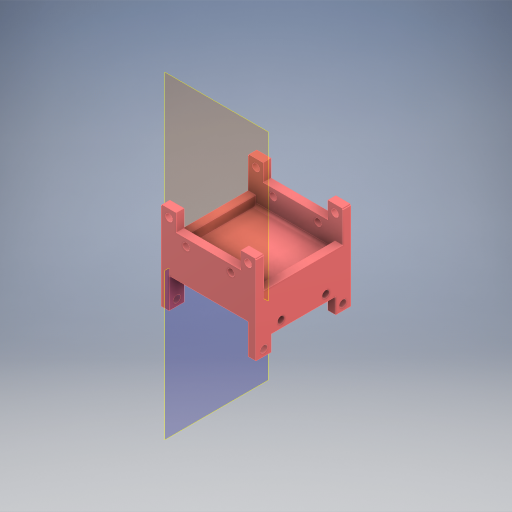
# Autodesk Inventor part: arm connection
Saved by Autodesk Inventor 2024 (Build 280153000, 153)
## iProperties
Created: 2024-09-08
Part Number: arm connection
Material: PMMA 플라스틱
Document SubType Name: Modeling
Designer: msi
Density: 1.188 g/cm^3
Appearance: 매끄러움 - 빨간색
Author: msi
Autodesk Inventor part; units mm, degrees
ref_plane "YZ Plane" through (0, 0, 0) normal (1, 0, 0) x (0, 1, 0)
ref_plane "XZ Plane" through (0, 0, 0) normal (0, 1, 0) x (-1, 0, 0)
ref_plane "XY Plane" through (0, 0, 0) normal (0, 0, 1) x (1, 0, 0)
ref_plane "작업 평면2" through (0, 0, 0) normal (0, 0, 1) x (1, 0, 0)
sketch "스케치2" plane through (0, 0, 0) normal (0, 0, 1) x (1, 0, 0)
  line L0 (7.15, 10.1828) -> (7.15, 9)
  arc A0 (7.15, 9) -> (9.15, 7) centre (9.15, 9) ccw
  line L1 (9.15, 7) -> (11.2, 7)
  arc A1 (12.2, 6) -> (11.2, 7) centre (11.2, 6) ccw
  line L2 (12.2, 6) -> (12.2, -27)
  arc A2 (11.2, -28) -> (12.2, -27) centre (11.2, -27) ccw
  line L3 (11.2, -28) -> (9.15, -28)
  arc A3 (9.15, -28) -> (7.15, -30) centre (9.15, -30) ccw
  line L4 (7.15, -30) -> (7.15, -32)
  arc A4 (6.15, -33) -> (7.15, -32) centre (6.15, -32) ccw
  line L5 (6.15, -33) -> (-6.15, -33)
  arc A5 (-7.15, -32) -> (-6.15, -33) centre (-6.15, -32) ccw
  line L6 (-7.15, -32) -> (-7.15, -30)
  arc A6 (-7.15, -30) -> (-9.15, -28) centre (-9.15, -30) ccw
  line L7 (-9.15, -28) -> (-11.2, -28)
  arc A7 (-12.2, -27) -> (-11.2, -28) centre (-11.2, -27) ccw
  line L8 (-12.2, -27) -> (-12.2, 6)
  arc A8 (-11.2, 7) -> (-12.2, 6) centre (-11.2, 6) ccw
  line L9 (-11.2, 7) -> (-9.15, 7)
  arc A9 (-9.15, 7) -> (-7.15, 9) centre (-9.15, 9) ccw
  line L10 (-7.15, 9) -> (-7.15, 10.1828)
  spline S0 degree 3 poles (-7.15, 10.1828) (-7.15, 10.4656) (-7.1021, 10.8015) (-6.9309, 11.2744) (-6.801, 11.5043) (-6.5407, 11.7954) (-6.3826, 11.9196) (-6.2267, 12) knots 0 0 0 0 0.420045 0.420045 0.746892 0.746892 1 1 1 1
  line L11 (-12.7, 12) -> (-6.2267, 12)
  line L12 (-17.8, 6) -> (-12.7, 12)
  line L13 (-17.8, -32.6) -> (-17.8, 6)
  line L14 (-12.7, -38.6) -> (-17.8, -32.6)
  line L15 (12.7, -38.6) -> (-12.7, -38.6)
  line L16 (17.8, -32.6) -> (12.7, -38.6)
  line L17 (17.8, 6) -> (17.8, -32.6)
  line L18 (12.7, 12) -> (17.8, 6)
  line L19 (6.2267, 12) -> (12.7, 12)
  spline S1 degree 3 poles (6.2267, 12) (6.3826, 11.9196) (6.5407, 11.7954) (6.801, 11.5043) (6.9309, 11.2744) (7.1021, 10.8015) (7.15, 10.4656) (7.15, 10.1828) knots 0 0 0 0 0.253108 0.253108 0.579955 0.579955 1 1 1 1
  circle A10 centre (15, 4.5) radius 1.35
  circle A11 centre (15, -12.5) radius 1.35
  circle A12 centre (8.5, -35.8) radius 1.35
  circle A13 centre (-15, 4.5) radius 1.35
  circle A14 centre (-15, -12.5) radius 1.35
  circle A15 centre (-8.5, -35.8) radius 1.35
  circle A16 centre (15, -29.5) radius 1.35
  circle A17 centre (-15, -29.5) radius 1.35
  line L20 (12.3, -27) -> (12.3, 6)
  arc A18 (12.3, 6) -> (11.2, 7.1) centre (11.2, 6) ccw
  line L21 (11.2, 7.1) -> (9.15, 7.1)
  arc A19 (7.25, 9) -> (9.15, 7.1) centre (9.15, 9) ccw
  line L22 (7.25, 9) -> (7.25, 10.1828)
  line L23 (6.5559, 11.9) -> (12.6538, 11.9)
  line L24 (12.6538, 11.9) -> (17.7, 5.9632)
  line L25 (17.7, 5.9632) -> (17.7, -32.5632)
  line L26 (-17.7, -32.5632) -> (-17.7, 5.9632)
  line L27 (-17.7, 5.9632) -> (-12.6538, 11.9)
  line L28 (-12.6538, 11.9) -> (-6.5559, 11.9)
  line L29 (-7.25, 10.1828) -> (-7.25, 9)
  arc A20 (-9.15, 7.1) -> (-7.25, 9) centre (-9.15, 9) ccw
  line L30 (-9.15, 7.1) -> (-11.2, 7.1)
  arc A21 (-11.2, 7.1) -> (-12.3, 6) centre (-11.2, 6) ccw
  line L31 (-12.3, 6) -> (-12.3, -27)
  arc A22 (-12.3, -27) -> (-11.2, -28.1) centre (-11.2, -27) ccw
  line L32 (-11.2, -28.1) -> (-9.15, -28.1)
  arc A23 (-7.25, -30) -> (-9.15, -28.1) centre (-9.15, -30) ccw
  line L33 (-7.25, -30) -> (-7.25, -32)
  arc A24 (-7.25, -32) -> (-6.15, -33.1) centre (-6.15, -32) ccw
  line L34 (-6.15, -33.1) -> (6.15, -33.1)
  arc A25 (6.15, -33.1) -> (7.25, -32) centre (6.15, -32) ccw
  line L35 (7.25, -32) -> (7.25, -30)
  arc A26 (9.15, -28.1) -> (7.25, -30) centre (9.15, -30) ccw
  line L36 (9.15, -28.1) -> (11.2, -28.1)
  arc A27 (11.2, -28.1) -> (12.3, -27) centre (11.2, -27) ccw
  line L37 (-12.3, -27) -> (-17.7, -27)
  line L38 (-17.7, -27) -> (-17.7, -38.5)
  line L39 (-12.3, -33.1) -> (-12.3, -27)
  line L40 (-12.3, -33.1) -> (12.2, -33.1)
  line L41 (17.7, -32.5632) -> (12.3, -32.5632)
  line L42 (12.3, -32.5632) -> (12.3, -26.5632)
  line L43 (12.3, -26.5632) -> (17.7, -26.5632)
  line L44 (17.7, -26.5632) -> (17.7, -32.5632)
  line L45 (17.7, -32.5632) -> (17.7, -38.5)
  line L46 (12.3, -32.4727) -> (12.3, -33.1)
  line L47 (12.2, -33.1) -> (12.3, -33.1)
  line L48 (17.7, -38.5) -> (17.7, -38.6)
  line L49 (17.7, -38.6) -> (-17.7, -38.6)
  line L50 (-17.7, -38.6) -> (-17.7, -38.5)
  line L51 (-17.7, -38.6) -> (17.7, -38.6)
  line L52 (17.7, -38.6) -> (17.7, -43.6)
  line L53 (17.7, -43.6) -> (-17.7, -43.6)
  line L54 (-17.7, -43.6) -> (-17.7, -38.6)
  line L55 (-17.7, -43.6) -> (17.7, -43.6)
  line L56 (17.7, -43.6) -> (17.7, -48.6)
  line L57 (17.7, -48.6) -> (-17.7, -48.6)
  line L58 (-17.7, -48.6) -> (-17.7, -43.6)
  spline S2 degree 5 poles (7.25, 10.1828) (7.25, 10.3319) (7.2395, 10.4809) (7.2209, 10.6292) (7.1668, 10.9238) (7.0686, 11.2074) (7.0011, 11.3424) (6.8856, 11.5458) (6.7393, 11.7287) (6.6819, 11.7898) (6.6205, 11.8469) (6.5559, 11.9) knots 0 0 0 0 0 0 0.3898 0.3898 0.3898 0.781377 0.781377 0.781377 1 1 1 1 1 1
  spline S3 degree 5 poles (-6.5559, 11.9) (-6.6205, 11.8469) (-6.6819, 11.7898) (-6.7393, 11.7287) (-6.8856, 11.5458) (-7.0011, 11.3424) (-7.0686, 11.2074) (-7.1668, 10.9238) (-7.2209, 10.6292) (-7.2395, 10.4809) (-7.25, 10.3319) (-7.25, 10.1828) knots 0 0 0 0 0 0 0.218623 0.218623 0.218623 0.6102 0.6102 0.6102 1 1 1 1 1 1
  point P0 (0, 0)
  point P1 (-6.15, -33.1)
  dimension "d1" = 0.1
  dimension "d3" = 6
  dimension "d4" = 5
  dimension "d7" = 5
  constraints: 78 end point, 21 point on circle, 12 parallel, 10 centre point, 6 horizontal, 5 perpendicular, 2 point on line, 1 vertical, 29 other
  measures "d1" distance between parallel lines of L2 L20
  measures "d3" distance of L41.end L42.end
  measures "d4" distance of L51.end L52.end
  measures "d7" distance of L55.end L56.end
extrude "돌출2" add sketch "스케치2" along normal blind 3 contours L45 L48 L49 L16 | L16 L15 L14 L38 L26 L37 L39 L40 L34 L47 L46 L41 L45 | L49 L52 L53 L54 L15 | L41 L42 L20 L43 L25 | L49 L50 L38 L14 | L56 L57 L58 L53
sketch "스케치4" plane through (0, 0, 0) normal (0, 0, -1) x (-1, 0, 0)
  line L0 (17.7, -48.6) -> (-17.7, -48.6) projected
  line L1 (17.7, -27) -> (17.7, -48.6) projected
  line L2 (12.3, -27) -> (17.7, -27) projected
  line L3 (12.3, -33.1) -> (12.3, -27) projected
  line L4 (-12.3, -33.1) -> (12.3, -33.1) projected
  line L5 (-12.3, -26.5632) -> (-12.3, -33.1) projected
  line L6 (-17.7, -26.5632) -> (-12.3, -26.5632) projected
  line L7 (-17.7, -48.6) -> (-17.7, -26.5632) projected
  circle A0 centre (-15, -29.5) radius 1.35 projected
  circle A1 centre (15, -29.5) radius 1.35 projected
  circle A2 centre (-8.5, -35.8) radius 1.35 projected
  circle A3 centre (8.5, -35.8) radius 1.35 projected
  line L8 (-17.7, -42.1) -> (17.7, -42.1)
  line L9 (17.7, -42.1) -> (17.7, -45.1)
  line L10 (17.7, -45.1) -> (-17.7, -45.1)
  line L11 (-17.7, -45.1) -> (-17.7, -42.1)
  line L12 (-17.7, -42.1) -> (17.7, -45.1) construction
  line L13 (17.7, -42.1) -> (-17.7, -45.1) construction
  point P0 (0, 0)
  point P1 (0, -43.6)
  dimension "d10" = 3
  constraints: 12 end point, 2 midpoint, 2 parallel, 1 horizontal, 1 perpendicular, 1 point on line
  measures "d10" distance of L8.end L9.end
extrude "돌출3" add sketch "스케치4" along normal blind 15 contours L10 L7 L8 L1
mirror "미러1" about plane through (0, -43.6, -15) normal (0, 0, -1)
ref_plane "작업 평면3" through (-15, -87.2, -15) normal (-1, 0, 0) x (0, 0, -1)
sketch "스케치5" plane through (-15, -87.2, -15) normal (-1, 0, 0) x (0, 0, -1)
  line L0 (-12.7, 12) -> (-9.2, 12) projected
  line L1 (-12.7, 12) -> (-17.8, 6) projected
  line L2 (-17.8, 6) -> (-17.8, -32.6) projected
  line L3 (-17.8, -32.6) -> (-12.7, -38.6) projected
  line L4 (-12.7, -38.6) -> (12.7, -38.6) projected
  line L5 (12.7, -38.6) -> (17.8, -32.6) projected
  line L6 (17.8, -32.6) -> (17.8, 6) projected
  line L7 (17.8, 6) -> (12.7, 12) projected
  line L8 (9.2, 12) -> (12.7, 12) projected
  arc A0 (12.2, 9) -> (9.2, 12) centre (9.2, 9) ccw projected
  line L9 (12.2, -30) -> (12.2, 9) projected
  arc A1 (9.2, -33) -> (12.2, -30) centre (9.2, -30) ccw projected
  line L10 (-9.2, -33) -> (9.2, -33) projected
  arc A2 (-12.2, -30) -> (-9.2, -33) centre (-9.2, -30) ccw projected
  line L11 (-12.2, 9) -> (-12.2, -30) projected
  arc A3 (-9.2, 12) -> (-12.2, 9) centre (-9.2, 9) ccw projected
  circle A4 centre (-15, 4.5) radius 1.35 projected
  circle A5 centre (-15, -12.5) radius 1.35 projected
  circle A6 centre (-8.5, -35.8) radius 1.35 projected
  circle A7 centre (15, 4.5) radius 1.35 projected
  circle A8 centre (15, -12.5) radius 1.35 projected
  circle A9 centre (8.5, -35.8) radius 1.35 projected
  circle A10 centre (-15, -29.5) radius 1.35 projected
  circle A11 centre (15, -29.5) radius 1.35 projected
  line L12 (-15, -42.1) -> (15, -42.1) projected
  line L13 (-15, -60.2) -> (-15, -45.1) projected
  line L14 (-15, -45.1) -> (15, -45.1) projected
  line L15 (15, -60.2) -> (15, -45.1) projected
  line L16 (15, -60.2) -> (18, -60.2) projected
  line L17 (18, -60.2) -> (18, -38.6) projected
  line L18 (15, -38.6) -> (18, -38.6) projected
  line L19 (15, -42.1) -> (15, -38.6) projected
  line L20 (-15, -42.1) -> (15, -42.1) projected
  line L21 (-15, -42.1) -> (-15, -38.6) projected
  line L22 (-15, -38.6) -> (-18, -38.6) projected
  line L23 (-18, -60.2) -> (-18, -38.6) projected
  line L24 (-15, -60.2) -> (-18, -60.2) projected
  line L25 (-15, -42.1) -> (-15, -38.6) projected
  line L26 (18, -60.2) -> (18, -38.6) projected
  line L27 (12.3, -30) -> (12.3, 9)
  arc A12 (12.3, 9) -> (10.2954, 11.9) centre (9.2, 9) ccw
  line L28 (10.2954, 11.9) -> (12.6538, 11.9)
  line L29 (12.6538, 11.9) -> (17.7, 5.9632)
  line L30 (17.7, 5.9632) -> (17.7, -27.1)
  line L31 (-17.7, -27.1) -> (-17.7, 5.9632)
  line L32 (-17.7, 5.9632) -> (-12.6538, 11.9)
  line L33 (-12.6538, 11.9) -> (-10.2954, 11.9)
  arc A13 (-10.2954, 11.9) -> (-12.3, 9) centre (-9.2, 9) ccw
  line L34 (-12.3, 9) -> (-12.3, -30)
  arc A14 (-12.3, -30) -> (-9.2, -33.1) centre (-9.2, -30) ccw
  line L35 (-9.2, -33.1) -> (9.2, -33.1)
  arc A15 (9.2, -33.1) -> (12.3, -30) centre (9.2, -30) ccw
  line L36 (15, -38.6) -> (-15, -38.6)
  line L37 (-15, -38.6) -> (-15, -33.1)
  line L38 (-15, -33.1) -> (15, -33.1)
  line L39 (15, -33.1) -> (15, -38.6)
  line L40 (18, -38.6) -> (15, -38.6)
  line L41 (15, -38.6) -> (15, -33.1)
  line L42 (15, -33.1) -> (18, -33.1)
  line L43 (18, -33.1) -> (18, -38.6)
  line L44 (18, -33.1) -> (12.3, -33.1)
  line L45 (12.3, -33.1) -> (12.3, -27.1)
  line L46 (12.3, -27.1) -> (18, -27.1)
  line L47 (18, -27.1) -> (18, -33.1)
  line L48 (-18, -38.6) -> (-15, -38.6)
  line L49 (-15, -38.6) -> (-15, -33.1)
  line L50 (-15, -33.1) -> (-18, -33.1)
  line L51 (-18, -33.1) -> (-18, -38.6)
  line L52 (-18, -33.1) -> (-12.3, -33.1)
  line L53 (-12.3, -33.1) -> (-12.3, -27.1)
  line L54 (-12.3, -27.1) -> (-18, -27.1)
  line L55 (-18, -27.1) -> (-18, -33.1)
  point P0 (-15, -87.2)
  point P1 (12.3, -30)
  point P2 (12.3, -33.1)
  point P3 (9.2, -33.1)
  point P4 (-9.2, -33.1)
  point P5 (-12.3, -33.1)
  point P6 (-12.3, -30)
  point P7 (-15, -38.6)
  point P8 (-12.7, -38.6)
  point P9 (12.7, -38.6)
  dimension "d13" = 0.1
  dimension "d14" = 6
  dimension "d15" = 6
  constraints: 58 end point, 10 parallel, 8 point on circle, 5 horizontal, 5 perpendicular, 4 centre point, 4 point on line, 9 other
  measures "d13" radial gap between concentric circles of A1 A15
  measures "d14" distance of L44.end L45.end
  measures "d15" distance of L53.end L52.end
extrude "돌출4" add sketch "스케치5" along normal blind 3 contours L54 L34 L53 L38 L50 L3 L2 | L2 L3 L50 L55 L54 | L50 L37 L3 | L3 L37 L22 L51 L50 | L37 L38 L35 L39 L5 L4 L3 | L3 L36 L37 | L5 L39 L36 | L39 L42 L5 | L5 L42 L43 L18 L39 | L27 L46 L6 L5 L42 L38 L45 | L5 L6 L46 L47 L42
sketch "스케치6" plane through (-18, -87.2, -15) normal (-1, 0, 0) x (0, 0, 1)
  line L0 (-12.7, 38.6) -> (-17.8, 32.6) projected
  line L1 (-18, 38.6) -> (-18, 27.1) projected
  line L2 (-18, 27.1) -> (-12.3, 27.1) projected
  line L3 (-12.3, 27.1) -> (-12.3, 33.1) projected
  line L4 (-12.3, 33.1) -> (12.3, 33.1) projected
  line L5 (12.3, 33.1) -> (12.3, 27.1) projected
  line L6 (12.3, 27.1) -> (18, 27.1) projected
  line L7 (18, 27.1) -> (18, 38.6) projected
  line L8 (18, 38.6) -> (-18, 38.6) projected
  circle A0 centre (8.5, 35.8) radius 1.35 projected
  circle A1 centre (-8.5, 35.8) radius 1.35 projected
  circle A2 centre (15, 29.5) radius 1.35 projected
  circle A3 centre (-15, 29.5) radius 1.35 projected
  line L9 (15, 60.2) -> (15, 45.1) projected
  line L10 (15, 45.1) -> (-15, 45.1) projected
  line L11 (-15, 60.2) -> (-15, 45.1) projected
  line L12 (-15, 60.2) -> (-18, 60.2) projected
  line L13 (-18, 60.2) -> (-18, 38.6) projected
  line L14 (-15, 38.6) -> (-18, 38.6) projected
  line L15 (-15, 42.1) -> (-15, 38.6) projected
  line L16 (15, 42.1) -> (-15, 42.1) projected
  line L17 (15, 42.1) -> (15, 38.6) projected
  line L18 (15, 38.6) -> (18, 38.6) projected
  line L19 (18, 60.2) -> (18, 38.6) projected
  line L20 (15, 60.2) -> (18, 60.2) projected
  line L21 (-18, 38.6) -> (18, 38.6)
  line L22 (18, 38.6) -> (18, 42.1)
  line L23 (18, 42.1) -> (-18, 42.1)
  line L24 (-18, 42.1) -> (-18, 38.6)
  point P0 (15, 87.2)
  point P1 (15, 42.1)
  point P2 (-15, 42.1)
  point P3 (-18, 42.1)
  constraints: 8 end point, 2 parallel, 1 horizontal, 1 perpendicular, 1 point on line
extrude "돌출5" add sketch "스케치6" against normal blind 3 contours L13 L23 L15 L8 | L15 L16 L17 L8 | L17 L23 L19 L8
sketch "스케치7" plane through (-17.7, -27, 0) normal (-1, 0, 0) x (0, 0, 1)
  line L0 (-33, -18.1) -> (3, -18.1) projected
  line L1 (3, 0) -> (3, -18.1) projected
  line L2 (0, 0) -> (3, 0) projected
  line L3 (0, 0) -> (0, -15.1) projected
  line L4 (0, -15.1) -> (-30, -15.1) projected
  line L5 (-30, 0) -> (-30, -15.1) projected
  line L6 (-30, 0) -> (-33, 0) projected
  line L7 (-33, 0) -> (-33, -18.1) projected
  line L8 (-33, 0) -> (-30, 0)
  line L9 (-30, 0) -> (-30, -15.1)
  line L10 (-30, -15.1) -> (-33, -15.1)
  line L11 (-33, -15.1) -> (-33, 0)
  line L12 (0, 0) -> (3, 0)
  line L13 (3, 0) -> (3, -15.1)
  line L14 (3, -15.1) -> (0, -15.1)
  line L15 (0, -15.1) -> (0, 0)
  line L16 (-33, -15.1) -> (3, -15.1)
  line L17 (3, -15.1) -> (3, -18.1)
  line L18 (3, -18.1) -> (-33, -18.1)
  line L19 (-33, -18.1) -> (-33, -15.1)
  point P0 (0, 27)
  constraints: 24 end point, 6 parallel, 3 horizontal, 3 perpendicular, 2 point on line
extrude "돌출6" add sketch "스케치7" along normal blind 0.3
mirror "미러4" about plane through (0, 0, 0) normal (1, 0, 0)
fillet "모깎기1" radius 1 2 edges at (15, -45.1, -15) (-15, -45.1, -15)
sketch "스케치9" plane through (-18, -42.1, 0) normal (0, 1, 0) x (1, 0, 0)
  line L0 (0, 30) -> (36, 30) projected
  line L1 (0, 0) -> (0, 30) projected
  line L2 (36, 0) -> (0, 0) projected
  line L3 (36, 0) -> (36, 30) projected
  line L4 (0, 0) -> (3, 0)
  line L5 (3, 0) -> (3, 30)
  line L6 (3, 30) -> (0, 30)
  line L7 (0, 30) -> (0, 0)
  line L8 (36, 0) -> (33, 0)
  line L9 (33, 0) -> (33, 30)
  line L10 (33, 30) -> (36, 30)
  line L11 (36, 30) -> (36, 0)
  point P0 (18, 0)
  dimension "d24" = 3
  dimension "d25" = 30
  dimension "d26" = 3
  constraints: 16 end point, 4 parallel, 2 horizontal, 2 perpendicular, 1 point on line
  measures "d24" distance of L6.end L5.end
  measures "d25" distance of L5.end L4.end
  measures "d26" distance of L9.end L10.end
extrude "돌출7" add sketch "스케치9" along normal blind 3.5 contours L0 L5 L2 L1 | L0 L3 L2 L9
fillet "모깎기3" radius 1 2 edges at (0, -42.1, 0) (0, -42.1, -30)
